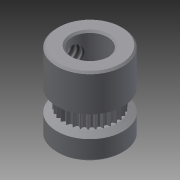
# Autodesk Inventor part: pinch wheel
Saved by Autodesk Inventor 2014 (Build 180170000, 170)
## iProperties
Created: 2013-12-11
Part Number: pinch wheel
Material: Generic
Document SubType Name: Modeling
Designer: caleb
Density: 1 g/cm^3
Appearance: Default
Author: caleb
Autodesk Inventor part; units mm, degrees
ref_plane "XY Plane" through (0, 0, 0) normal (0, 0, 1) x (1, 0, 0)
sketch "Sketch1" plane through (0, 0, 0) normal (0, 0, 1) x (1, 0, 0)
  circle A0 centre (0, 0) radius 4.7
  dimension "d0" = 9.4
  constraints: 1 centre point, 1 coincident
  measures "d0" diameter of A0
extrude "Extrusion1" add sketch "Sketch1" along normal blind 11
sketch "Sketch2" plane through (0, 0, 11) normal (0, 0, 1) x (1, 0, 0)
  circle A0 centre (0, 0) radius 4.7 projected
  circle A1 centre (0, 0) radius 2.5
  dimension "d3" = 5
  constraints: 1 centre point, 1 coincident
  measures "d3" diameter of A1
extrude "Extrusion2" cut sketch "Sketch2" against normal through all contours A1
ref_plane "Work Plane1" through (0, 0, 4.3) normal (0, 0, 1) x (1, 0, 0)
sketch "Sketch7" plane through (0, 0, 0) normal (1, 0, 0) x (0, 1, 0)
  line L0 (-6.58, 4.3) -> (6.58, 4.3) projected
  line L1 (-4.7, 0) -> (-4.7, 11) projected
  line L2 (-4.7, 5.8255) -> (-3.7899, 5.3)
  line L3 (-3.7899, 5.3) -> (-3.7899, 3.3)
  line L4 (-3.7899, 3.3) -> (-4.7, 2.7745)
  line L5 (0, -2.176) -> (0, 13.056) projected
  point P0 (0, 0)
  point P1 (-3.7899, 4.3)
  dimension "d22" = 30
  dimension "d23" = 30
  dimension "d24" = 2
  dimension "d25" = 3.7899
  constraints: 6 end point, 3 point on line, 1 midpoint, 1 parallel
  measures "d22" angle of L0 L4
  measures "d23" angle of L2 L0
  measures "d24" distance of L2.end L3.end
  measures "d25" distance from line of point (0, 0) L3
revolve "Revolution1" cut sketch "Sketch7" angle 360 about axis through (0, 0, -10) along (0, 0, 1)
sketch "Sketch4" plane through (0, 0, 0) normal (1, 0, 0) x (0, 1, 0)
  line L0 (-2.5, 11) -> (2.5, 11) construction
  line L1 (0, 8.4127) -> (0, 11) construction
  line L2 (0, 8.4127) -> (0, 5.8255) construction
  line L3 (4.7, 5.8255) -> (-4.7, 5.8255) construction
  point P0 (0, 0)
  constraints: 4 end point, 2 coincident, 2 midpoint, 1 collinear, 1 vertical alignment
hole "Hole1" at (0, 0, 8.4127) direction (-1, 0, 0) diameter 2.642 end through all thread size "6-32 UNC" class "2B" standard "ANSI Unified Screw Threads"
chamfer "Chamfer1" distance 0.25 angle 45 4 edges at (-4.7, 0, 11) (-4.7, 0, 0) (-2.5, 0, 0) (-2.5, 0, 11)
ref_plane "Work Plane3" through (0, -3.7899, 4.8) normal (0, -1, 0) x (1, 0, 0)
sketch "Sketch8" plane through (0, 0, 4.3) normal (0, 0, 1) x (1, 0, 0)
  circle A0 centre (0, 0) radius 3.7899 construction
  line L0 (-0.3572, 3.773) -> (-0.136, 3.3899)
  line L1 (-0.136, 3.3899) -> (0.136, 3.3899)
  line L2 (0.136, 3.3899) -> (0.3572, 3.773)
  arc A1 (0.3572, 3.773) -> (-0.3572, 3.773) centre (0, 0) ccw
  dimension "d30" = 120
  dimension "d31" = 120
  dimension "d32" = 0.7144
  dimension "d33" = 0.4
  constraints: 6 end point, 4 point on circle, 1 centre point, 1 concentric, 1 horizontal, 1 horizontal alignment
  measures "d30" angle of L1 L0
  measures "d31" angle of L2 L1
  measures "d32" distance of L2.end L0.start
  measures "d33" distance edge to line of A0 L1
extrude "Extrusion5" cut sketch "Sketch8" along normal mid plane 2
fillet "Fillet1" radius 0.05 4 edges at (-0.3572, 3.773, 4.3) (-0.136, 3.3899, 4.3) (0.3572, 3.773, 4.3) (0.136, 3.3899, 4.3)
sketch "Sketch6" plane through (-4.65, 0, 0) normal (-1, 0, 0) x (0, -1, 0)
  line L0 (-4.65, 10.88) -> (4.65, 10.88)
  line L1 (4.65, 10.88) -> (4.65, 6.2)
  line L2 (4.65, 6.2) -> (-4.65, 6.2)
  line L3 (-4.65, 6.2) -> (-4.65, 10.88)
  line L4 (4.65, 5.2) -> (-4.65, 5.2) projected
  line L5 (4.65, 10.88) -> (-4.65, 10.88) projected
  point P0 (0, 0)
  point P1 (0, 10.88)
  dimension "d18" = 1
  dimension "d19" = 9.4
  constraints: 8 end point, 2 parallel, 1 collinear, 1 horizontal, 1 midpoint, 1 perpendicular, 1 vertical alignment, 1 other
  measures "d18" distance between parallel lines of L4 L2
pattern_circular "Circular Pattern1" count 30 over 360 about axis through (0, 0, 0) along (0, 0, 1) of "Extrusion5", "Fillet1"
equation "\"d0\" = outer_diameter"
equation "\"d1\" = length"
equation "\"d3\" = shaft_diameter"
equation "\"d4\" = length"
equation "\"d24\" = hobbing_width"
equation "\"d25\" = 0.5 * pinch_diameter"
equation "\"d34\" = hobbing_width"
equation "\"d19\" = outer_diameter"
equation "\"outer_diameter\" = 9.4"
equation "\"shaft_diameter\" = 5"
equation "\"tap_thread_pitch\" = 0.79375"
equation "\"pi\" = 3.141593"
equation "\"length\" = 11"
equation "\"hobbing_offset\" = 4.3"
equation "\"d6\" = -hobbing_offset"
equation "\"hobbing_width\" = 2"
equation "\"setscrew_offset\" = 3"
equation "\"pinch_diameter\" = 7.579754"
body "Solid1"
